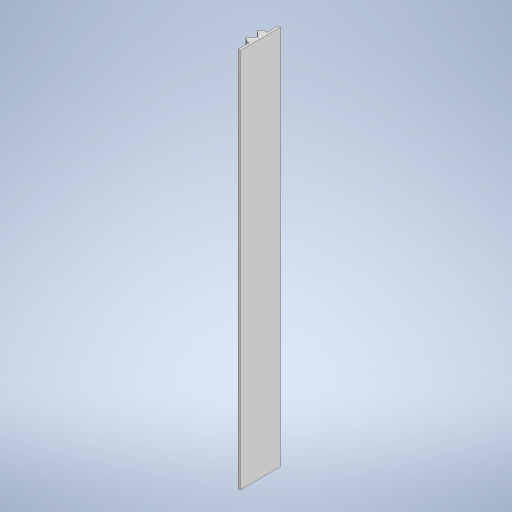
# Autodesk Inventor part: RailDerzavka
Saved by Autodesk Inventor 2024 (Build 280153000, 153)
## iProperties
Created: 2023-08-21
Part Number: RailDerzavka
Material: Generic
Document SubType Name: Modeling
Designer: KirikDK
Density: 1 g/cm^3
Appearance: Default
Author: KirikDK
Autodesk Inventor part; units mm, degrees
ref_plane "YZ Plane" through (0, 0, 0) normal (1, 0, 0) x (0, 1, 0)
ref_plane "XZ Plane" through (0, 0, 0) normal (0, 1, 0) x (-1, 0, 0)
ref_plane "XY Plane" through (0, 0, 0) normal (0, 0, 1) x (1, 0, 0)
sketch "Sketch1" plane through (0, 0, 0) normal (0, 1, 0) x (-1, 0, 0)
  line L0 (6, 5) -> (0, 5)
  line L1 (0, 5) -> (0, -5)
  line L2 (0, -5) -> (6, -5)
  line L3 (6, -5) -> (6, 5)
  line L4 (6, 5) -> (0, 0)
  line L5 (0, 0) -> (6, -5)
  line L6 (6, -5) -> (0, -10)
  line L7 (0, 18) -> (-2, 18)
  line L8 (-2, 18) -> (-2, -18)
  line L9 (-2, -18) -> (0, -18)
  line L10 (0, -18) -> (0, 18)
  line L11 (6, 5) -> (0, 10)
  point P0 (0, -10)
  point P1 (0, -5)
  point P2 (0, 5)
  constraints: 24 end point, 4 parallel, 2 horizontal, 2 perpendicular, 1 coincident, 1 point on line
extrude "Extrusion1" add sketch "Sketch1" along normal blind 340 contours L4 L1 L0 | L0 L10 L11 | L1 L10 L9 L8 L7 | L6 L10 L2 | L2 L1 L5
chamfer "Chamfer1" distance 0.1 angle 45 2 edges at (-6, 170, -5) (-6, 170, 5)
chamfer "Chamfer2" distance 1 angle 45 1 edges at (0, 170, 0)
sketch "Sketch2" plane through (0, 340, 0) normal (0, 1, 0) x (1, 0, 0)
  line L0 (-4, 12) -> (0, 12)
  line L1 (0, 12) -> (0, 8)
  line L2 (0, 8) -> (-4, 8)
  line L3 (-4, 8) -> (-4, 12)
  line L4 (-4, -12) -> (0, -12)
  line L5 (0, -12) -> (0, -8)
  line L6 (0, -8) -> (-4, -8)
  line L7 (-4, -8) -> (-4, -12)
  point P0 (0, 0)
  constraints: 16 end point, 4 parallel, 2 horizontal, 2 perpendicular, 1 point on line
extrude "Extrusion2" cut sketch "Sketch2" against normal blind 1000
body "Solid1"
